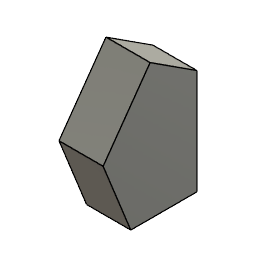
replay (Autodesk Fusion 360 design; units mm, degrees)
Autodesk Fusion 360 part; units mm, degrees
ref_plane "工作平面1" through (12, 0, 0) normal (1, 0, 0) x (0, 1, 0)
sketch "草图1" plane through (12, 0, 0) normal (1, 0, 0) x (0, 0, -1)
  line L0 (-7, 23) -> (-24, 34)
  line L1 (-24, 34) -> (-41, 10)
  line L2 (-41, 10) -> (-31, -15)
  line L3 (-31, -15) -> (-7, -15)
  line L4 (-7, -15) -> (-7, 23)
extrude "拉伸1" add sketch "草图1" along normal blind 16
